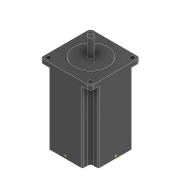
# Autodesk Inventor part: motor
Saved by Autodesk Inventor 2022 (Build 260153000, 153)
## iProperties
Created: 2022-03-21
Part Number: motor
Material: Generic
Document SubType Name: Sheet Metal
Designer: ferna
Density: 1 g/cm^3
Sheet Metal Rule: Default_mm
Appearance: Dark Gray
Mass: 244.496 g
Surface Area: 254.232 cm^2
Volume: 244.496 cm^3
Author: ferna
Autodesk Inventor part; units mm, degrees
ref_plane "YZ Plane" through (0, 0, 0) normal (1, 0, 0) x (0, 1, 0)
ref_plane "XZ Plane" through (0, 0, 0) normal (0, 1, 0) x (-1, 0, 0)
ref_plane "XY Plane" through (0, 0, 0) normal (0, 0, 1) x (1, 0, 0)
sketch "Sketch1" plane through (0, 0, 0) normal (0, 1, 0) x (-1, 0, 0)
  line L0 (3, 0) -> (54.2, 0)
  line L1 (56.2, -2) -> (56.2, -53.2)
  line L2 (53.2, -56.2) -> (3, -56.2)
  line L3 (0, -53.2) -> (0, -3)
  line L4 (56.2, 0) -> (51.7, 0)
  line L5 (51.7, 0) -> (51.7, -4.5)
  line L6 (51.7, -4.5) -> (56.2, -4.5)
  line L7 (56.2, -4.5) -> (56.2, 0)
  circle A0 centre (51.7, -4.5) radius 2.5
  line L8 (56.2, -56.2) -> (51.7, -56.2)
  line L9 (51.7, -56.2) -> (51.7, -51.7)
  line L10 (51.7, -51.7) -> (56.2, -51.7)
  line L11 (56.2, -51.7) -> (56.2, -56.2)
  circle A1 centre (51.7, -51.7) radius 2.5
  line L12 (0, 0) -> (4.5, 0)
  line L13 (4.5, 0) -> (4.5, -4.5)
  line L14 (4.5, -4.5) -> (0, -4.5)
  line L15 (0, -4.5) -> (0, 0)
  circle A2 centre (4.5, -4.5) radius 2.5
  circle A3 centre (4.5, -51.7) radius 2.5
  arc A4 (56.2, -2) -> (54.2, 0) centre (54.2, -2) ccw
  arc A5 (53.2, -56.2) -> (56.2, -53.2) centre (53.2, -53.2) ccw
  arc A6 (0, -53.2) -> (3, -56.2) centre (3, -53.2) ccw
  arc A7 (3, 0) -> (0, -3) centre (3, -3) ccw
  line L16 (51.7, -4.5) -> (4.5, -51.7)
  line L17 (4.5, -4.5) -> (51.7, -51.7)
  circle A8 centre (28.1, -28.1) radius 19
  point P0 (0, -56.2)
  dimension "d0" = 56.2
  dimension "d1" = 56.2
  dimension "d2" = 4.5
  dimension "d3" = 4.5
  dimension "d4" = 5
  dimension "d5" = 4.5
  dimension "d6" = 4.5
  dimension "d7" = 2
  dimension "d8" = 3
  dimension "d9" = 38
  dimension "d34" = 4.5
  dimension "d35" = 4.5
  constraints: 36 end point, 9 centre point, 9 point on line, 8 parallel, 8 point on circle, 8 tangent, 5 perpendicular, 4 coincident, 4 horizontal, 2 equal radius, 1 midpoint
  measures "d0" distance of L8.start point (0, -56.2)
  measures "d1" distance of L4.start L8.start
  measures "d2" distance of L6.end L5.end
  measures "d3" distance of L5.end L4.end
  measures "d4" diameter of A0
  measures "d5" distance of L8.end L9.end
  measures "d6" distance of L13.end L14.end
  measures "d7" radius of A4
  measures "d8" radius of A5
  measures "d9" diameter of A8
  measures "d34" distance from line of L2 L16.end
  measures "d35" distance from line of L0 L13.end
extrude "Extrusion1" add sketch "Sketch1" along normal blind 5 contours L0 L13 A2 L14 L3 A7 | L0 L5 A0 L16 A8 L17 A2 L13 | L0 A4 L1 L6 A0 L5 | L14 A2 L17 A8 A1 L9 L2 A6 L3 | L6 L1 L10 A1 L17 A8 L16 A0 | A8 L17 L16 | L16 L17 A8 | L17 L16 A8 | L9 A1 L10 L1 A5 L2 | L17 A8 L16
sketch "Sketch2" plane through (0, 5, 0) normal (0, 1, 0) x (1, 0, 0)
  circle A0 centre (-51.7, 4.5) radius 2.5 projected
  circle A1 centre (-4.5, 4.5) radius 2.5 projected
  circle A2 centre (-4.5, 51.7) radius 2.5 projected
  circle A3 centre (-51.7, 51.7) radius 2.5 projected
  circle A4 centre (-51.7, 4.5) radius 2.5 projected
  line L0 (-4.5, 51.7) -> (-4.5, 4.5)
  circle A5 centre (-27.7983, 28.3967) radius 19
  line L1 (-4.5, 4.5) -> (-14.6658, 14.6658)
  line L2 (-41.5292, 41.5292) -> (-51.7, 51.7)
  line L3 (-51.7, 4.5) -> (-28.25, 27.95)
  line L4 (-14.3658, 41.8342) -> (-4.5, 51.7)
  point P0 (0, 0)
  dimension "d12" = 38
  constraints: 10 end point, 4 perpendicular, 3 point on circle, 1 centre point, 1 vertical
  measures "d12" diameter of A5
extrude "Extrusion2" add sketch "Sketch2" along normal blind 1 contours A5
sketch "Sketch3" plane through (-27.7983, 6, -28.3967) normal (0, 1, 0) x (1, 0, 0)
  circle A0 centre (0, 0) radius 3.2
  circle A1 centre (0, 0) radius 3.05
  line L0 (-3.05, 0) -> (-3.05, 0.9682)
  line L1 (-3.05, 0) -> (-3.05, -0.9682)
  point P0 (27.7983, -28.3967)
  dimension "d16" = 6.1
  dimension "d15" = 6.4
  constraints: 4 end point, 2 point on circle, 2 vertical, 1 centre point, 1 coincident, 1 horizontal alignment, 1 point on line, 2 other
  measures "d15" diameter of A0
extrude "Extrusion3" add sketch "Sketch3" along normal blind 20 contours A1 | A0 L1 L0 picked at (-2.904, -1.0385)
sketch "Sketch4" plane through (0, 0, 0) normal (0, -1, 0) x (1, 0, 0)
  line L0 (-3, -56.2) -> (-53.2, -56.2) projected
  line L1 (-56.2, -53.2) -> (-56.2, -2) projected
  line L2 (-54.2, 0) -> (-3, 0) projected
  line L3 (0, -3) -> (0, -53.2) projected
  arc A0 (-56.2, -53.2) -> (-53.2, -56.2) centre (-53.2, -53.2) ccw projected
  line L4 (-56.2, -2) -> (-56.2, 0)
  arc A1 (-54.2, 0) -> (-56.2, -2) centre (-54.2, -2) ccw projected
  line L5 (-56.2, 0) -> (-54.2, 0)
  line L6 (-3, 0) -> (0, 0)
  arc A2 (0, -3) -> (-3, 0) centre (-3, -3) ccw projected
  line L7 (0, 0) -> (0, -3)
  arc A3 (-3, -56.2) -> (0, -53.2) centre (-3, -53.2) ccw projected
  line L8 (-3, -56.2) -> (0, -56.2)
  line L9 (0, -56.2) -> (0, -53.2)
  circle A4 centre (-51.7, -51.7) radius 2.5 projected
  line L10 (-53.2, -56.2) -> (-47.2, -56.2)
  line L11 (-47.2, -55.2) -> (-47.2, -50.2)
  line L12 (-50.2, -47.2) -> (-55.2, -47.2)
  line L13 (-56.2, -47.2) -> (-56.2, -53.2)
  line L14 (-56.2, -56.2) -> (-47.2, -47.2) construction
  line L15 (-47.2, -56.2) -> (-56.2, -47.2) construction
  arc A5 (-47.2, -50.2) -> (-50.2, -47.2) centre (-50.2, -50.2) ccw
  arc A6 (-56.2, -53.2) -> (-53.2, -56.2) centre (-53.2, -53.2) ccw
  circle A7 centre (-51.7, -4.5) radius 2.5 projected
  circle A8 centre (-4.5, -4.5) radius 2.5 projected
  circle A9 centre (-4.5, -51.7) radius 2.5 projected
  line L16 (-55.2, -9) -> (-50.2, -9)
  line L17 (-47.2, -6) -> (-47.2, -1)
  line L18 (-47.2, 0) -> (-56.2, 0)
  line L19 (-56.2, 0) -> (-56.2, -9)
  circle A10 centre (-51.7, -4.5) radius 2.5 projected
  line L20 (-56.2, -9) -> (-47.2, 0) construction
  line L21 (-47.2, -9) -> (-56.2, 0) construction
  line L22 (-6, -9) -> (-1, -9)
  line L23 (0, -9) -> (0, 0)
  line L24 (0, 0) -> (-9, 0)
  line L25 (-9, -1) -> (-9, -6)
  line L26 (-9, -9) -> (0, 0) construction
  line L27 (0, -9) -> (-9, 0) construction
  line L28 (-9, -56.2) -> (0, -56.2)
  line L29 (0, -56.2) -> (0, -47.2)
  line L30 (-1, -47.2) -> (-6, -47.2)
  line L31 (-9, -50.2) -> (-9, -55.2)
  line L32 (-9, -56.2) -> (0, -47.2) construction
  line L33 (0, -56.2) -> (-9, -47.2) construction
  arc A11 (-50.2, -9) -> (-47.2, -6) centre (-50.2, -6) ccw
  arc A12 (-9, -6) -> (-6, -9) centre (-6, -6) ccw
  arc A13 (-6, -47.2) -> (-9, -50.2) centre (-6, -50.2) ccw
  line L34 (-46.2, -56.2) -> (-10, -56.2)
  line L35 (-3, -56.2) -> (-53.2, -56.2) projected
  line L36 (-56.2, -46.2) -> (-56.2, -10)
  line L37 (-54.2, 0) -> (-3, 0) projected
  line L38 (-46.2, 0) -> (-10, 0)
  line L39 (0, -10) -> (0, -46.2)
  arc A14 (-56.2, -46.2) -> (-55.2, -47.2) centre (-55.2, -46.2) ccw
  arc A15 (-47.2, -55.2) -> (-46.2, -56.2) centre (-46.2, -55.2) ccw
  arc A16 (-55.2, -9) -> (-56.2, -10) centre (-55.2, -10) ccw
  arc A17 (-46.2, 0) -> (-47.2, -1) centre (-46.2, -1) ccw
  arc A18 (-9, -1) -> (-10, 0) centre (-10, -1) ccw
  arc A19 (0, -10) -> (-1, -9) centre (-1, -10) ccw
  arc A20 (-1, -47.2) -> (0, -46.2) centre (-1, -46.2) ccw
  arc A21 (-10, -56.2) -> (-9, -55.2) centre (-10, -55.2) ccw
  point P0 (-56.2, -47.2)
  point P1 (-46.9, -55.9)
  point P2 (-9, -55.9)
  point P3 (-46.9, 0)
  point P4 (-55.9, -9)
  point P5 (-55.9, -46.9)
  point P6 (0, -46.2)
  point P7 (-56.2, -10)
  point P8 (-46.2, 0)
  point P9 (-56.2, -46.2)
  dimension "d19" = 9
  dimension "d20" = 9
  dimension "d21" = 3
  dimension "d22" = 9
  dimension "d23" = 9
  dimension "d24" = 3
  dimension "d27" = 1
  constraints: 68 end point, 29 tangent, 28 point on line, 26 point on circle, 13 centre point, 10 equal radius, 8 midpoint, 8 parallel, 7 perpendicular, 6 horizontal, 2 collinear
  measures "d19" distance of L13.start L14.end
  measures "d20" distance of L14.end L10.end
  measures "d21" radius of A5
  measures "d22" distance of L18.end L18.start
  measures "d23" distance of L18.start L21.start
  measures "d24" radius of A11
  measures "d27" radius of A14
extrude "Extrusion4" add sketch "Sketch4" along normal blind 80 contours L0 A15 L11 A5 L12 A14 L1 A16 L16 A11 L17 A17 L2 A18 L25 A12 L22 A19 L3 A20 L30 A13 L31 A21
sketch "Sketch5" plane through (-56.2, 0, -2) normal (-1, 0, 0) x (0, 0, 1)
  line L0 (-44.2, 0) -> (-44.2, -80) projected
  line L1 (-44.2, -80) -> (-26.1, -80)
  line L2 (-8, -80) -> (-44.2, -80) projected
  line L3 (-26.1, -80) -> (-26.1, -75)
  line L4 (-20.1, -80) -> (-32.1, -80)
  line L5 (-32.1, -80) -> (-32.1, -70)
  line L6 (-32.1, -70) -> (-20.1, -70)
  line L7 (-20.1, -70) -> (-20.1, -80)
  line L8 (-20.1, -80) -> (-32.1, -70) construction
  line L9 (-32.1, -80) -> (-20.1, -70) construction
  point P0 (2, 0)
  dimension "d28" = 18.1
  dimension "d29" = 5
  dimension "d30" = 12
  dimension "d31" = 10
  constraints: 16 end point, 3 midpoint, 2 parallel, 2 perpendicular, 1 horizontal
  measures "d28" distance of L0.end L1.end
  measures "d29" distance of L1.end L3.end
  measures "d30" distance of L5.end L6.end
  measures "d31" distance of L4.end L5.end
extrude "Extrusion5" add sketch "Sketch5" along normal blind 1
sketch "Sketch6" plane through (0, 5, 0) normal (0, 1, 0) x (1, 0, 0)
  circle A0 centre (-27.7983, 28.3967) radius 19 projected
  arc A1 (-53.2, 56.2) -> (-56.2, 53.2) centre (-53.2, 53.2) ccw projected
  line L0 (-56.2, 53.2) -> (-56.2, 2) projected
  arc A2 (-56.2, 2) -> (-54.2, 0) centre (-54.2, 2) ccw projected
  line L1 (-54.2, 0) -> (-3, 0) projected
  arc A3 (-3, 0) -> (0, 3) centre (-3, 3) ccw projected
  line L2 (0, 3) -> (0, 53.2) projected
  arc A4 (0, 53.2) -> (-3, 56.2) centre (-3, 53.2) ccw projected
  line L3 (-3, 56.2) -> (-53.2, 56.2) projected
  circle A5 centre (-4.5, 51.7) radius 2.5 projected
  circle A6 centre (-51.7, 51.7) radius 2.5 projected
  circle A7 centre (-4.5, 4.5) radius 2.5 projected
  circle A8 centre (-51.7, 4.5) radius 2.5 projected
  point P0 (0, 0)
sketch "Sketch7" plane through (-54.2, 5, 0) normal (0, 0, 1) x (1, 0, 0)
  line L0 (44.2, -85) -> (8, -85) projected
  line L1 (26.1, -85) -> (26.1, -82)
  circle A0 centre (26.1, -82) radius 3
  point P0 (54.2, -5)
  dimension "d36" = 3
  constraints: 2 end point, 1 centre point, 1 coincident, 1 midpoint, 1 tangent, 1 vertical
  measures "d36" distance of L1.start L1.end
sketch "Sketch8" plane through (0, 0, -53.2) normal (1, 0, 0) x (0, 0, -1)
  line L0 (-7, -80) -> (-43.2, -80) projected
  line L1 (-25.1, -80) -> (-25.1, -77)
  circle A0 centre (-25.1, -77) radius 3
  point P0 (-53.2, 0)
  dimension "d37" = 3
  constraints: 2 end point, 1 coincident, 1 midpoint, 1 vertical, 1 vertical alignment, 2 other
  measures "d37" distance of L1.start L1.end
equation "\"BendRadius\" = Thickness"
equation "\"BendReliefWidth\" = Thickness"
equation "\"BendReliefDepth\" = 0.5 * Thickness"
equation "\"CornerReliefSize\" = 4 * Thickness"
equation "\"MinimumRemnant\" = 2 * Thickness"
equation "\"TransitionRadius\" = BendRadius"
equation "\"JacobiRadiusSize\" = BendRadius"
equation "\"GapSize\" = Thickness"
equation "\"Thickness\" = 0.5"
body "Solid1"
